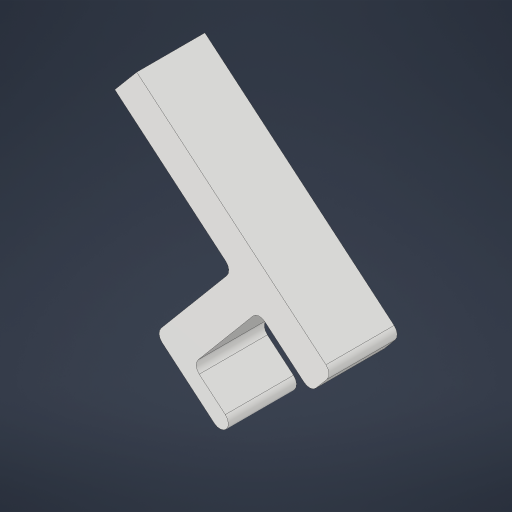
# Autodesk Inventor part: CL4-015
Saved by Autodesk Inventor 2023.4 (Build 274418000, 418)
## iProperties
Created: 2025-02-08
Part Number: CL4-015
Material: ABS Plastic
Document SubType Name: Modeling
Designer: brand
Density: 1.06 g/cm^3
Appearance: Smooth - White
Author: brand
Autodesk Inventor part; units mm, degrees
ref_plane "YZ Plane" through (0, 0, 0) normal (1, 0, 0) x (0, 1, 0)
ref_plane "XZ Plane" through (0, 0, 0) normal (0, 1, 0) x (-1, 0, 0)
ref_plane "XY Plane" through (0, 0, 0) normal (0, 0, 1) x (1, 0, 0)
sketch "Sketch1" plane through (0, 0, 0) normal (0, 0, 1) x (1, 0, 0)
  line L0 (0, 127) -> (76.2, 127) construction
  line L1 (76.2, 127) -> (76.2, 0) construction
  line L2 (76.2, 0) -> (0, 0) construction
  line L3 (0, 0) -> (0, 127) construction
  line L4 (107.95, 80.9498) -> (293.751, 80.9498) construction
  line L5 (107.95, 80.9498) -> (293.751, 80.9498) construction
  line L6 (293.751, 80.9498) -> (293.751, 61.8998) construction
  line L7 (293.751, 61.8998) -> (107.95, 61.8998) construction
  line L8 (107.95, 61.8998) -> (107.95, 80.9498) construction
  line L9 (66.5231, 143.6203) -> (139.4888, 82.3948)
  line L10 (139.4888, 82.3948) -> (147.6522, 92.1236)
  line L11 (147.6522, 92.1236) -> (74.6865, 153.3491)
  line L12 (91.4594, 64.6709) -> (120.0313, 98.7216)
  line L13 (91.4594, 64.6709) -> (81.7306, 72.8343)
  line L14 (81.7306, 72.8343) -> (110.3025, 106.885)
  line L15 (91.4594, 64.6709) -> (106.0525, 52.4258)
  line L16 (106.0525, 52.4258) -> (110.1342, 57.2902)
  line L17 (110.1342, 57.2902) -> (95.5411, 69.5353)
  line L18 (74.6865, 153.3491) -> (66.5231, 143.6203)
  point P0 (107.95, 71.4248)
  dimension "d0" = 127
  dimension "d1" = 76.2
  dimension "d2" = 46.0502
  dimension "d3" = 185.801
  dimension "d4" = 19.05
  dimension "d5" = 31.75
  dimension "d6" = 12.7
  dimension "d7" = 12.7
  dimension "d8" = 25.4
  dimension "d9" = 44.45
  dimension "d11" = 19.05
  dimension "d13" = 6.35
  dimension "d14" = 50
  dimension "d15" = 95.25
  constraints: 38 end point, 11 perpendicular, 4 parallel, 3 horizontal, 3 point on line, 1 coincident, 1 midpoint, 1 other
  measures "d0" distance of L0.end L1.end
  measures "d1" distance of L1.end L2.end
  measures "d2" distance between parallel lines of L4 L0
  measures "d3" distance of L4.start L4.end
  measures "d4" distance of L4.end L6.end
  measures "d5" distance from line of point (107.95, 71.425) L1
  measures "d6" distance of L9.end L10.end
  measures "d7" distance of L12.start L13.end
  measures "d8" distance between parallel lines of L10 L12
  measures "d9" distance of L12.start L12.end
  measures "d11" distance of L12.start L15.end
  measures "d13" distance of L15.end L16.end
  measures "d14" angle of L9 L1
  measures "d15" distance of L10.end L11.end
extrude "Extrusion1" add sketch "Sketch1" against normal blind 25.4
fillet "Fillet1" radius 3.175 8 edges at (95.5411, 69.5353, -12.7) (120.0313, 98.7216, -12.7) (139.4888, 82.3948, -12.7) (147.6522, 92.1236, -12.7) (110.3025, 106.885, -12.7) (106.0525, 52.4258, -12.7) (110.1342, 57.2902, -12.7) (81.7306, 72.8343, -12.7)
body "Solid1"
